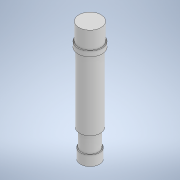
# Autodesk Inventor part: celestronFinder
Saved by Autodesk Inventor 2021.1 (Build 251245000, 245)
## iProperties
Created: 2020-07-29
Part Number: celestronFinder
Material: Generic
Document SubType Name: Modeling
Designer: robst
Density: 1 g/cm^3
Appearance: Default
Author: robst
Autodesk Inventor part; units mm, degrees
ref_plane "YZ Plane" through (0, 0, 0) normal (1, 0, 0) x (0, 1, 0)
ref_plane "XZ Plane" through (0, 0, 0) normal (0, 1, 0) x (-1, 0, 0)
ref_plane "XY Plane" through (0, 0, 0) normal (0, 0, 1) x (1, 0, 0)
sketch "Sketch1" plane through (0, 0, 0) normal (0, 0, 1) x (1, 0, 0)
  line L0 (0, 0) -> (-13.97, 0)
  line L1 (-13.97, 0) -> (-13.97, -21.844)
  line L2 (-13.97, -21.844) -> (-15.24, -21.844)
  line L3 (-15.24, -21.844) -> (-15.24, -28.194)
  line L4 (-15.24, -28.194) -> (-13.1445, -28.194)
  line L5 (-13.1445, -28.194) -> (-13.1445, -115.824)
  line L6 (-13.1445, -115.824) -> (-10.7315, -115.824)
  line L7 (-10.7315, -115.824) -> (-10.7315, -137.668)
  line L8 (-10.7315, -137.668) -> (-11.938, -137.668)
  line L9 (-11.938, -137.668) -> (-11.938, -150.368)
  line L10 (-11.938, -150.368) -> (0, -150.368)
  line L11 (0, -150.368) -> (0, 0)
  dimension "d0" = 21.844
  dimension "d1" = 13.97
  dimension "d2" = 6.35
  dimension "d3" = 15.24
  dimension "d4" = 13.1445
  dimension "d5" = 87.63
  dimension "d7" = 10.7315
  dimension "d8" = 21.844
  dimension "d9" = 11.938
  dimension "d10" = 12.7
  constraints: 24 end point, 6 perpendicular, 5 horizontal, 1 vertical
  measures "d0" distance of L0.end L1.end
  measures "d1" distance from line of L1 L0.start
  measures "d2" distance of L2.end L3.end
  measures "d3" distance from line of L3 L0.start
  measures "d4" distance from line of L5 L0.start
  measures "d5" vertical distance of L5.end L3.end
  measures "d7" distance from line of L7 L0.start
  measures "d8" distance of L7.end L6.end
  measures "d9" distance from line of L0.start L9
  measures "d10" distance of L9.end L8.end
revolve "Revolution1" add sketch "Sketch1" angle 360 about axis through (0, -150.368, 0) along (0, 1, 0)
equation "\"d0\" = endLength"
equation "\"d1\" = endRadius"
equation "\"d2\" = bandLength"
equation "\"d3\" = bandRadius"
equation "\"d4\" = mainBodyRadius"
equation "\"d5\" = mainBodyLength"
equation "\"d7\" = eyepieceEndRadius"
equation "\"d8\" = endLength"
equation "\"d9\" = eyepieceRadius"
equation "\"d10\" = eyepieceLength"
equation "\"endRadius\" = 13.97"
equation "\"bandRadius\" = 15.24"
equation "\"mainBodyRadius\" = 13.1445"
equation "\"eyepieceEndRadius\" = 10.7315"
equation "\"eyepieceRadius\" = 11.938"
equation "\"endLength\" = 21.844"
equation "\"bandLength\" = 6.35"
equation "\"mainBodyLength\" = 87.63"
equation "\"eyepieceEndLength\" = 13.97"
equation "\"eyepieceLength\" = 12.7"
body "Solid1"
